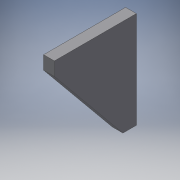
# Autodesk Inventor part: Fianchi supp.saldato
Saved by Autodesk Inventor 2018 (Build 220112000, 112)
## iProperties
Created: 2020-06-01
Part Number: Fianchi supp.saldato
Material: Generico
Document SubType Name: Modeling
Designer: Francesco
Density: 1 g/cm^3
Appearance: Default
Author: Francesco
Autodesk Inventor part; units mm, degrees
ref_plane "YZ Plane" through (0, 0, 0) normal (1, 0, 0) x (0, 1, 0)
ref_plane "XZ Plane" through (0, 0, 0) normal (0, 1, 0) x (-1, 0, 0)
ref_plane "XY Plane" through (0, 0, 0) normal (0, 0, 1) x (1, 0, 0)
sketch "Schizzo1" plane through (0, 0, 0) normal (1, 0, 0) x (0, 1, 0)
  line L0 (0, 0) -> (61, 0)
  line L1 (61, 0) -> (61, -72)
  line L2 (61, -72) -> (51, -72)
  line L3 (0, 0) -> (0, -10)
  line L4 (0, -10) -> (51, -72)
  dimension "d0" = 61
  dimension "d1" = 72
  dimension "d2" = 10
  dimension "d3" = 10
  constraints: 10 end point, 2 perpendicular, 1 horizontal, 1 vertical
  measures "d0" distance of L0.start L0.end
  measures "d1" distance of L0.end L1.end
  measures "d2" distance of L1.end L2.end
  measures "d3" distance of L0.start L3.end
extrude "Estrusione1" add sketch "Schizzo1" along normal blind 8
